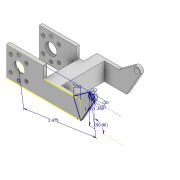
# Autodesk Inventor part: Odometry holder for metal drive train
Saved by Autodesk Inventor 2020 (Build 240168000, 168)
## iProperties
Created: 2020-03-04
Part Number: Odometry holder for metal drive train
Material: Generic
Document SubType Name: Modeling
Designer: ball
Density: 1 g/cm^3
Appearance: Default
Author: ball
Autodesk Inventor part; units mm, degrees
ref_plane "YZ Plane" through (0, 0, 0) normal (1, 0, 0) x (0, 1, 0)
ref_plane "XZ Plane" through (0, 0, 0) normal (0, 1, 0) x (-1, 0, 0)
ref_plane "XY Plane" through (0, 0, 0) normal (0, 0, 1) x (1, 0, 0)
sketch "Sketch1" plane through (0, 0, 0) normal (0, 1, 0) x (-1, 0, 0)
  line L0 (10.16, 20.955) -> (-21.59, 20.955)
  line L1 (-21.59, 20.955) -> (-21.59, 18.415)
  line L2 (-21.59, 18.415) -> (10.16, 18.415)
  line L3 (10.16, 18.415) -> (10.16, 20.955)
  line L4 (10.16, -6.985) -> (-21.59, -6.985)
  line L5 (-21.59, -6.985) -> (-21.59, -9.525)
  line L6 (-21.59, -9.525) -> (10.16, -9.525)
  line L7 (10.16, -9.525) -> (10.16, -6.985)
  point P0 (0, 0)
  dimension "d0" = 31.75
  dimension "d1" = 2.54
  dimension "d2" = 10.16
  dimension "d3" = 20.955
  dimension "d4" = 31.75
  dimension "d5" = 2.54
  dimension "d6" = 10.16
  dimension "d7" = 30.48
  constraints: 16 end point, 4 parallel, 2 horizontal, 2 perpendicular
  measures "d0" distance of L2.end L1.end
  measures "d1" distance of L1.end L0.end
  measures "d2" distance from line of L3 point (0, 0)
  measures "d3" distance from line of L0 point (0, 0)
  measures "d4" distance of L6.end L5.end
  measures "d5" distance of L5.end L4.end
  measures "d6" distance from line of L7 point (0, 0)
  measures "d7" distance between parallel lines of L6 L0
extrude "Extrusion1" add sketch "Sketch1" along normal blind 25.4
sketch "Sketch2" plane through (0, 0, 0) normal (0, 1, 0) x (-1, 0, 0)
  line L0 (-21.59, 18.415) -> (10.16, 18.415) projected
  line L1 (10.16, -6.985) -> (-21.59, -6.985) projected
  line L2 (-21.59, 18.415) -> (-34.29, 18.415)
  line L3 (10.16, 18.415) -> (10.16, 20.955) projected
  line L4 (-21.59, -9.525) -> (-25.4, -9.525)
  line L5 (-21.59, -6.985) -> (-21.59, -9.525) projected
  line L6 (-21.59, -9.525) -> (-21.59, 18.415)
  line L7 (-25.4, -9.525) -> (-25.4, -20.955)
  line L8 (-25.4, -20.955) -> (-34.29, -20.955)
  line L9 (-34.29, -20.955) -> (-34.29, 18.415)
  line L10 (-21.59, 18.415) -> (10.16, 18.415) projected
  line L11 (10.16, -9.525) -> (10.16, -6.985) projected
  line L12 (10.16, 20.955) -> (-21.59, 20.955) projected
  point P0 (0, 0)
  point P1 (-21.59, -6.985)
  dimension "d16" = 35.56
  dimension "d17" = 41.91
  dimension "d18" = 12.7
  constraints: 12 end point, 1 collinear, 1 horizontal, 1 perpendicular, 1 point on line, 1 vertical
  measures "d16" distance between parallel lines of L7 L11
  measures "d17" distance between parallel lines of L8 L12
  measures "d18" distance between parallel lines of L9 L6
extrude "Extrusion2" add sketch "Sketch2" along normal blind 15.24
sketch "Sketch4" plane through (0, 0, 0) normal (0, 1, 0) x (-1, 0, 0)
  line L0 (-34.29, -20.955) -> (-25.4, -20.955) projected
  line L1 (-34.29, -20.955) -> (-53.34, -20.955)
  line L2 (-53.34, -20.955) -> (-53.34, -18.415)
  line L3 (-53.34, -18.415) -> (-34.29, -18.415)
  line L4 (-34.29, -18.415) -> (-34.29, -20.955)
  line L5 (-21.59, 20.955) -> (-53.34, 20.955)
  line L6 (-53.34, 20.955) -> (-53.34, 18.415)
  line L7 (-53.34, 18.415) -> (-21.59, 18.415)
  line L8 (-21.59, 18.415) -> (-21.59, 20.955)
  line L9 (10.16, 18.415) -> (10.16, 20.955) projected
  line L10 (10.16, -9.525) -> (10.16, -6.985) projected
  point P0 (0, 0)
  point P1 (-50.8, -18.415)
  dimension "d20" = 2.54
  dimension "d24" = 2.54
  dimension "d55" = 63.5
  dimension "d56" = 63.5
  constraints: 16 end point, 4 parallel, 2 horizontal, 2 perpendicular, 1 point on line
  measures "d20" distance of L1.end L2.end
  measures "d24" distance of L6.end L5.end
  measures "d55" distance between parallel lines of L9 L6
  measures "d56" distance between parallel lines of L10 L2
extrude "Extrusion3" add sketch "Sketch4" along normal blind 15.24
sketch "Sketch5" plane through (-10.16, 25.4, 20.955) normal (0, 0, 1) x (1, 0, 0)
  circle A0 centre (10.16, -12.7) radius 4.8895
  line L0 (0, -25.4) -> (0, 0) projected
  line L1 (-16.3, -25.4) -> (92.4658, -25.4) projected
  circle A1 centre (10.16, -22.225) radius 1.397
  circle A2 centre (16.8952, -19.4352) radius 1.397
  circle A3 centre (19.685, -12.7) radius 1.397
  circle A4 centre (16.8952, -5.9648) radius 1.397
  circle A5 centre (10.16, -3.175) radius 1.397
  circle A6 centre (3.4248, -5.9648) radius 1.397
  circle A7 centre (0.635, -12.7) radius 1.397
  circle A8 centre (3.4248, -19.4352) radius 1.397
  point P0 (10.16, -25.4)
  dimension "d26" = 9.779
  dimension "d27" = 10.16
  dimension "d28" = 12.7
  dimension "d29" = 2.794
  dimension "d30" = 9.525
  dimension "d33" = 360
  constraints: 9 centre point, 17 other
  measures "d26" diameter of A0
  measures "d27" distance from line of L0 A0.centre
  measures "d28" distance from line of L1 A0.centre
  measures "d29" diameter of A1
  measures "d30" distance of A1.centre A0.centre
extrude "Extrusion4" cut sketch "Sketch5" against normal through all contours A0 | A1 | A2 | A4 | A5 | A6 | A8
sketch "Sketch6" plane through (-10.16, 25.4, 20.955) normal (0, 0, 1) x (1, 0, 0)
  circle A0 centre (72.3186, -3.302) radius 2.2
  circle A1 centre (10.16, -12.7) radius 4.8895 construction
  line L0 (0, 0) -> (31.75, 0) construction
  line L1 (75.6206, -25.4) -> (75.6206, 0) construction
  line L2 (75.6206, -25.4) -> (101.0206, -25.4) construction
  arc A2 (75.1858, -4.9396) -> (70.3884, -0.6228) centre (72.3186, -3.302) ccw
  line L3 (63.5, -25.4) -> (44.45, -25.4) construction
  line L4 (75.1858, -4.9396) -> (98.796, -4.9396) construction
  line L5 (70.3884, -0.6228) -> (57.15, -10.16)
  line L6 (63.5, -10.16) -> (44.45, -10.16) construction
  line L7 (63.5, -25.4) -> (63.5, -10.16) construction
  line L8 (31.75, -10.16) -> (63.5, -10.16) projected
  line L9 (0, -25.4) -> (63.5, -25.4) projected
  line L10 (75.1858, -4.9396) -> (63.5, -25.4)
  line L11 (57.15, -10.16) -> (63.5, -25.4)
  point P0 (10.16, -25.4)
  point P1 (60.96, -25.4)
  point P2 (60.96, -10.16)
  dimension "d37" = 4.4
  dimension "d38" = 62.865
  dimension "d39" = 3.302
  dimension "d40" = 25.4
  dimension "d41" = 90
  dimension "d42" = 3.302
  dimension "d53" = 6.604
  dimension "d57" = 6.35
  constraints: 12 end point, 2 centre point, 2 horizontal, 2 point on circle, 2 tangent, 1 coincident, 1 perpendicular, 1 point on line, 1 vertical
  measures "d37" diameter of A0
  measures "d38" distance of A1.centre A0.centre
  measures "d39" distance from line of A0.centre L0
  measures "d40" distance of L1.start L1.end
  measures "d41" angle of L2 L1
  measures "d42" distance from line of A0.centre L1
  measures "d53" diameter of A2
  measures "d57" distance from line of L5.end L7
extrude "Extrusion8" add sketch "Sketch6" against normal blind 2.54
sketch "Sketch9" plane through (25.4, 0, -20.955) normal (0, 0, -1) x (-1, 0, 0)
  line L0 (-39.6182, 20.447) -> (-27.94, 0.2198) projected
  line L1 (-21.59, 15.24) -> (-34.8284, 24.7772) projected
  arc A0 (-34.8284, 24.7772) -> (-39.6258, 20.4604) centre (-36.7586, 22.098) ccw projected
  circle A1 centre (-36.7586, 22.098) radius 2.2 projected
  line L2 (-39.6258, 20.4604) -> (-27.94, 0) projected
  line L3 (-27.94, 0) -> (-8.89, 0) projected
  line L4 (-21.59, 15.24) -> (-27.94, 0)
  point P0 (25.4, 0)
  constraints: 2 end point
extrude "Extrusion10" add sketch "Sketch9" against normal blind 2.54
equation "\"d5\" = d1"
equation "\"d6\" = d2"
equation "\"d56\" = d55"
body "Solid1"
